Autodesk Fusion 360 part; units mm, degrees
(part 2 of 2)
  constraint parallel L233 L235
  constraint tangent A234 L235
  constraint tangent L234 A234
  constraint tangent A231 L232
  constraint tangent A231 L235
  constraint tangent L232 A232
  constraint tangent A232 L233
  constraint tangent L233 A233
  constraint tangent A233 L234
  constraint horizontal L236
  constraint perpendicular L236 L237
  constraint parallel L236 L238
  constraint parallel L237 L239
  constraint tangent A238 L239
  constraint tangent L238 A238
  constraint tangent A235 L236
  constraint tangent A235 L239
  constraint tangent L236 A236
  constraint tangent A236 L237
  constraint tangent L237 A237
  constraint tangent A237 L238
  constraint tangent L145 A239
  constraint tangent A239 L240
  constraint tangent L146 A240
  constraint tangent L240 A240
  constraint tangent L145 A241
  constraint tangent L241 A241
  constraint tangent L147 A242
  constraint tangent L241 A242
  constraint tangent L147 A243
  constraint tangent L242 A243
  constraint tangent L126 A244
  constraint tangent L242 A244
  constraint tangent L126 A245
  constraint tangent L243 A245
  constraint tangent L148 A246
  constraint tangent L243 A246
  constraint tangent L148 A247
  constraint tangent L244 A247
  constraint tangent L149 A248
  constraint tangent L244 A248
  constraint tangent L151 A249
  constraint tangent L245 A249
  constraint tangent L150 A250
  constraint tangent L245 A250
  constraint tangent A146 L246
  constraint tangent L151 A251
  constraint tangent L246 A251
  constraint tangent A145 L247
  constraint tangent L129 A252
  constraint tangent L247 A252
  constraint tangent L150 A253
  constraint tangent L248 A253
  constraint tangent L128 A254
  constraint tangent L248 A254
  measures "d1" diameter of A0
  measures "d2" diameter of A1
  measures "d3" diameter of A2
  measures "d4" diameter of A3
  measures "d5" diameter of A4
  measures "d9" diameter of A136
  measures "d12" diameter of A137
extrude "Extrude1" add sketch "mriya" along normal blind 10.5 contours L106 A111 A112 L107 A113 L108 A114 L109 A115 L110 A116 L111 A117 L112 A118 L113 L114 A120 L115 A121 L116 A122 L117 A123 L118 A124 L119 A125 L120 A126 L121 A127 L122 A128 L123 A129 L124 A130 L125 A131 L126 L127 A133 L128 L129 A134 L130 A135 L131 L132 L142 L143 A143 L144 A145 A146 L145 L146 L147 L148 L149 L150 L151 A239 L240 A240 L241 A241 A242 L242 A243 A244 L243 A245 A246 L244 A247 A248 L245 A249 A250 L246 A251 L247 A252 L248 A253 A254 makes body 1
extrude "Extrude2" add sketch "mriya" along normal blind 17 contours L113 A119 L114 A132 L127 L131 L132 L149 bodies 1
extrude "Extrude3" add sketch "mriya" along normal blind 2 from surface at 1.7 contours L106 A111 A112 L107 A113 L108 A114 L109 A115 L110 A116 L111 A117 L112 A118 L113 L114 A120 L115 A121 L116 A122 L117 A123 L118 A124 L119 A125 L120 A126 L121 A127 L122 A128 L123 A129 L124 A130 L125 A131 L133 L134 L135 L136 A138 A139 A140 L137 L138 L139 A141 A142 L142 L143 A143 | L113 A119 L114 L133 L134 L135 L136 A138 A139 A140 | L114 L137 L138 L139 A141 A142 | A147 | A148 | A149 | A150 bodies 1
extrude "Extrude6" add sketch "mriya" along normal blind 1 from surface at 14.3 contours L113 A119 L114 L133 L134 L135 L136 A138 A139 A140 bodies 1
extrude "Extrude7" add sketch "mriya" along normal blind 1 from surface at 7.8 contours L114 L137 L138 L139 A141 A142 bodies 1
chamfer "Chamfer2" distance 0.8 angle 45 4 edges at (-16.65, 78.0432, 14.3) (-7.05, 48.8432, 14.3) (-7.504, 77.5892, 14.3) (-7.05, 9.5932, 7.8) on bodies 1
sketch "power-switch" plane through (-4.55, 0, 0) normal (1, 0, 0) x (0, 1, 0)
  line L0 (1.9932, 0) -> (76.4932, 0)
  line L1 (76.4932, 0) -> (76.4932, 17)
  line L2 (76.4932, 17) -> (19.1932, 17)
  line L3 (19.1932, 17) -> (19.1932, 10.5)
  line L4 (19.1932, 10.5) -> (1.9932, 10.5)
  line L5 (1.9932, 10.5) -> (1.9932, 0)
  line L6 (35.9932, 5.2) -> (25.7932, 5.2)
  line L7 (25.7932, 5.2) -> (25.7932, 7.9)
  line L8 (25.7932, 7.9) -> (35.9932, 7.9)
  line L9 (35.9932, 7.9) -> (35.9932, 5.2)
  line L10 (37.1432, 3.05) -> (24.6432, 3.05)
  line L11 (23.6432, 4.05) -> (23.6432, 9.05)
  line L12 (24.6432, 10.05) -> (37.1432, 10.05)
  line L13 (38.1432, 9.05) -> (38.1432, 4.05)
  arc A0 (24.6432, 10.05) -> (23.6432, 9.05) centre (24.6432, 9.05) ccw
  arc A1 (38.1432, 9.05) -> (37.1432, 10.05) centre (37.1432, 9.05) ccw
  arc A2 (37.1432, 3.05) -> (38.1432, 4.05) centre (37.1432, 4.05) ccw
  arc A3 (23.6432, 4.05) -> (24.6432, 3.05) centre (24.6432, 4.05) ccw
  constraint perpendicular L6 L7
  constraint tangent L11 A0
  constraint tangent L12 A0
  constraint tangent L12 A1
  constraint tangent L13 A1
  constraint tangent L10 A2
  constraint tangent L13 A2
  constraint tangent L10 A3
  constraint tangent L11 A3
  constraint vertical L7
  constraint perpendicular L7 L8
  constraint vertical L9
extrude "Extrude8" cut sketch "power-switch" against normal blind 2.5 contours L6 L7 L8 L9 bodies 1
extrude "Extrude9" cut sketch "power-switch" against normal blind 1.2 contours L10 L11 L12 L13 A0 A1 A2 A3 bodies 1
fillet "Fillet10" radius 0.2 8 edges at (-4.55, 30.8932, 3.05) (-4.55, 23.9361, 3.3429) (-4.55, 23.6432, 6.55) (-4.55, 23.9361, 9.7571) (-4.55, 30.8932, 10.05) (-4.55, 37.8503, 9.7571) (-4.55, 38.1432, 6.55) (-4.55, 37.8503, 3.3429) on bodies 1
sketch "usb-c" plane through (0, 80.5432, 0) normal (0, 1, 0) x (-1, 0, 0)
  line L0 (3.6, 0) -> (36.1295, 0)
  line L1 (3.6, 16.7) -> (3.6, 0)
  line L2 (21.2002, 10.9) -> (21.2002, 10.1)
  arc A0 (21.2002, 10.9) -> (19.8003, 12.3) centre (19.8003, 10.9) ccw
  line L3 (11.8003, 10.1) -> (11.8003, 10.9)
  line L4 (19.8003, 8.7) -> (13.2003, 8.7)
  line L5 (19.7003, 7) -> (13.3002, 7)
  arc A1 (11.8003, 10.1) -> (13.2003, 8.7) centre (13.2003, 10.1) ccw
  line L6 (22.7003, 11) -> (22.7003, 10)
  line L7 (13.3002, 14) -> (19.7003, 14)
  arc A2 (13.2002, 12.3) -> (11.8002, 10.9) centre (13.2002, 10.9) ccw
  arc A3 (19.8003, 8.7) -> (21.2003, 10.1) centre (19.8003, 10.1) ccw
  line L8 (10.3002, 10) -> (10.3002, 11)
  line L9 (13.2002, 12.3) -> (19.8003, 12.3)
  line L10 (8.6, 0) -> (41.1295, 0)
  line L11 (41.1295, 10.5) -> (25.9, 10.5)
  line L12 (25.9, 10.5) -> (25.9, 17)
  line L13 (25.9, 17) -> (8.6, 17)
  line L14 (8.6, 17) -> (8.6, 0)
  line L15 (41.1295, 0) -> (41.1295, 10.5)
  arc A4 (13.3002, 14) -> (10.3002, 11) centre (13.3002, 11) ccw
  arc A5 (22.7003, 11) -> (19.7003, 14) centre (19.7003, 11) ccw
  arc A6 (10.3002, 10) -> (13.3002, 7) centre (13.3003, 10) ccw
  arc A7 (19.7003, 7) -> (22.7003, 10) centre (19.7003, 10) ccw
  constraint tangent L3 A2
  constraint tangent A2 L9
  constraint tangent A0 L9
  constraint tangent L2 A0
  constraint tangent L4 A3
  constraint tangent L2 A3
  constraint tangent L4 A1
  constraint tangent L3 A1
  constraint perpendicular L6 L7
  constraint perpendicular L5 L8
  constraint horizontal L5
  constraint perpendicular L5 L6
  constraint tangent L8 A4
  constraint tangent L7 A4
  constraint tangent L7 A5
  constraint tangent L6 A5
  constraint tangent L5 A6
  constraint tangent L8 A6
  constraint tangent L6 A7
  constraint tangent L5 A7
extrude "Extrude10" cut sketch "usb-c" against normal blind 2.5 contours L2 A0 L3 L4 A1 A2 A3 L9 bodies 1
extrude "Extrude11" cut sketch "usb-c" against normal blind 1.2 contours L5 L6 L7 L8 A4 A5 A6 A7 bodies 1
fillet "Fillet16" radius 0.2 8 edges at (-10.3002, 80.5432, 10.5) (-11.1789, 80.5432, 13.1213) (-16.5002, 80.5432, 14) (-21.8216, 80.5432, 13.1213) (-22.7003, 80.5432, 10.5) (-21.8216, 80.5432, 7.8787) (-16.5002, 80.5432, 7) (-11.1789, 80.5432, 7.8787) on bodies 1
fillet "Fillet19" radius 1 8 edges at (-5.75, 30.8932, 10.05) (-5.75, 37.8503, 9.7571) (-5.75, 38.1432, 6.55) (-5.75, 37.8503, 3.3429) (-5.75, 30.8932, 3.05) (-5.75, 23.9361, 3.3429) (-5.75, 23.6432, 6.55) (-5.75, 23.9361, 9.7571) on bodies 1
fillet "Fillet20" radius 1 8 edges at (-16.5002, 79.3432, 7) (-11.1789, 79.3432, 7.8787) (-10.3002, 79.3432, 10.5) (-11.1789, 79.3432, 13.1213) (-16.5002, 79.3432, 14) (-21.8216, 79.3432, 13.1213) (-22.7003, 79.3432, 10.5) (-21.8216, 79.3432, 7.8787) on bodies 1
fillet "Fillet21" radius 1 90 edges at (-33.5148, 80.5432, 10.5) (-41.5122, 80.6193, 10.5) (-42.4009, 81.4003, 10.5) (-43.9383, 82.6148, 10.5) (-51.508, 82.8432, 10.5) (-58.3122, 82.9193, 10.5) (-60.3009, 84.8003, 10.5) (-62.9383, 87.1148, 10.5) (-73.4, 87.3432, 10.5) (-83.8617, 87.1148, 10.5) (-85.9991, 85.3003, 10.5) (-87.4878, 83.9193, 10.5) (-94.792, 83.8432, 10.5) (-102.8617, 83.6148, 10.5) (-107.2491, 79.5503, 10.5) (-110.9878, 75.9193, 10.5) (-116.042, 75.8432, 10.5) (-121.8617, 75.6148, 10.5) (-123.3991, 74.4003, 10.5) (-124.2878, 73.6193, 10.5) (-131.3852, 73.5432, 10.5) (-140.9638, 72.357, 10.5) (-142.15, 42.8932, 10.5) (-140.9638, 13.4294, 10.5) (-120.4039, 12.2432, 10.5) (-100.9856, 12.5857, 10.5) (-96.4776, 16.6093, 10.5) (-92.7807, 20.091, 10.5) (-84.5771, 20.2432, 10.5) (-75.6268, 19.8342, 10.5) (-70.4599, 11.5202, 10.5) (-65.1097, 3.0203, 10.5) (-56.008, 2.5432, 10.5) (-48.2878, 2.4671, 10.5) (-47.3991, 1.6861, 10.5) (-45.8617, 0.4716, 10.5) (-37.192, 0.2432, 10.5) (-29.2878, 0.1671, 10.5) (-28.3991, -0.6139, 10.5) (-26.8617, -1.8284, 10.5) (-17.1568, -2.0568, 10.5) (-5.7362, -0.8706, 10.5) (-4.55, 10.5932, 10.5) (-4.55, 47.8432, 17) (-5.7362, 79.357, 17) (-17.25, 80.5432, 17) (-24.8648, 80.5432, 0) (-41.5122, 80.6193, 0) (-42.4009, 81.4003, 0) (-43.9383, 82.6148, 0) (-51.508, 82.8432, 0) (-58.3122, 82.9193, 0) (-60.3009, 84.8003, 0) (-62.9383, 87.1148, 0) (-73.4, 87.3432, 0) (-83.8617, 87.1148, 0) (-85.9991, 85.3003, 0) (-87.4878, 83.9193, 0) (-94.792, 83.8432, 0) (-102.8617, 83.6148, 0) (-107.2491, 79.5503, 0) (-110.9878, 75.9193, 0) (-116.042, 75.8432, 0) (-121.8617, 75.6148, 0) (-123.3991, 74.4003, 0) (-124.2878, 73.6193, 0) (-131.3852, 73.5432, 0) (-140.9638, 72.357, 0) (-142.15, 42.8932, 0) (-140.9638, 13.4294, 0) (-120.4039, 12.2432, 0) (-100.9856, 12.5857, 0) (-96.4776, 16.6093, 0) (-92.7807, 20.091, 0) (-84.5771, 20.2432, 0) (-75.6268, 19.8342, 0) (-70.4599, 11.5202, 0) (-65.1097, 3.0203, 0) (-56.008, 2.5432, 0) (-48.2878, 2.4671, 0) (-47.3991, 1.6861, 0) (-45.8617, 0.4716, 0) (-37.192, 0.2432, 0) (-29.2878, 0.1671, 0) (-28.3991, -0.6139, 0) (-26.8617, -1.8284, 0) (-17.1568, -2.0568, 0) (-5.7362, -0.8706, 0) (-4.55, 39.2432, 0) (-5.7362, 79.357, 0) on bodies 1
fillet "Fillet22" radius 0.5 6 edges at (-6.3, 19.1932, 17) (-4.8429, 19.1932, 16.7071) (-4.55, 19.1932, 12.75) (-25.9, 80.5432, 12.75) (-25.9, 80.2503, 16.7071) (-25.9, 78.7932, 17) on bodies 1
chamfer "Chamfer1" distance 0.5 angle 45 4 edges at (-7.05, 30.8932, 5.2) (-7.05, 35.9932, 6.55) (-7.05, 30.8932, 7.9) (-7.05, 25.7932, 6.55) on bodies 1
mirror "Mirror1" about plane through (0, 0, 0) normal (1, 0, 0) of bodies 1 makes body 2
named bodies: "Left", "Right"
